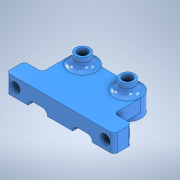
# Autodesk Inventor part: 4mm_Roller_Spacer
Saved by Autodesk Inventor 2021 (Build 250183000, 183)
## iProperties
Created: 2021-03-29
Part Number: 4mm_Roller_Spacer
Material: PET Plastic
Document SubType Name: Modeling
Designer: Jorian Brusind
Density: 1.541 g/cm^3
Appearance: Cyan
Author: Jorian Brusind
Autodesk Inventor part; units mm, degrees
ref_plane "YZ Plane" through (0, 0, 0) normal (1, 0, 0) x (0, 1, 0)
ref_plane "XZ Plane" through (0, 0, 0) normal (0, 1, 0) x (-1, 0, 0)
ref_plane "XY Plane" through (0, 0, 0) normal (0, 0, 1) x (1, 0, 0)
sketch "Sketch4" plane through (0, 0, 0) normal (0, 1, 0) x (-1, 0, 0)
  circle A0 centre (0, 0) radius 7.5
  circle A1 centre (0, 0) radius 2.75
  dimension "d19" = 15
  dimension "d20" = 5.5
  constraints: 2 centre point, 2 coincident
  measures "d19" diameter of A0
  measures "d20" diameter of A1
extrude "Extrusion4" add sketch "Sketch4" along normal blind 10
ref_plane "Work Plane2" through (0, 5, 0) normal (0, 1, 0) x (1, 0, 0)
sketch "Sketch12" plane through (0, 5, 0) normal (0, 1, 0) x (1, 0, 0)
  circle A0 centre (0, 0) radius 2.75 projected
  line L0 (0, 0) -> (25, 0)
  circle A1 centre (25, 0) radius 2.75
  circle A2 centre (25, 0) radius 7.5
  line L1 (12.5, 0) -> (12.5, -20)
  line L2 (42.5, -25) -> (-17.5, -25)
  line L3 (-17.5, -25) -> (-17.5, -15)
  line L4 (-17.5, -15) -> (42.5, -15)
  line L5 (42.5, -15) -> (42.5, -25)
  line L6 (42.5, -25) -> (-17.5, -15) construction
  line L7 (-17.5, -25) -> (42.5, -15) construction
  circle A3 centre (0, 0) radius 7.5 projected
  line L8 (18.6557, -4) -> (6.3443, -4)
  line L9 (6.3443, -4) -> (6.3443, 4)
  line L10 (6.3443, 4) -> (18.6557, 4)
  line L11 (18.6557, 4) -> (18.6557, -4)
  line L12 (18.6557, -4) -> (6.3443, 4) construction
  line L13 (6.3443, -4) -> (18.6557, 4) construction
  line L14 (6.3443, 4) -> (18.6557, 4)
  line L15 (18.6557, 4) -> (18.6557, -16)
  line L16 (18.6557, -16) -> (6.3443, -16)
  line L17 (6.3443, -16) -> (6.3443, 4)
  point P0 (6.3443, -15)
  point P1 (18.6557, -15)
  dimension "d66" = 25
  dimension "d67" = 5.5
  dimension "d68" = 15
  dimension "d69" = 20
  dimension "d70" = 60
  dimension "d71" = 10
  dimension "d72" = 8
  dimension "d73" = 20
  constraints: 36 end point, 6 parallel, 5 midpoint, 4 horizontal, 3 perpendicular, 2 centre point, 2 coincident, 1 vertical, 2 other
  measures "d66" distance of L0.start L0.end
  measures "d67" diameter of A1
  measures "d68" diameter of A2
  measures "d69" distance of L1.start L1.end
  measures "d70" distance of L3.end L4.end
  measures "d71" distance of L2.end L3.end
  measures "d72" distance of L8.end L9.end
  measures "d73" distance of L14.end L15.end
extrude "Extrusion10" add sketch "Sketch12" along normal mid plane 10 contours A3 L10 A2 L0 | L0 L1 L8 A3 | L0 A2 L8 L1 | L8 L1 L4 L17 | A2 L11 L0 | L0 L11 A2 | L8 L15 L4 L1 | A2 L11 | L17 L16 L15 L4 L5 L2 L3 | L4 L1 L16 L17 | L4 L15 L16 L1
sketch "Sketch13" plane through (18.6557, 10, -4) normal (0, 0, -1) x (-1, 0, 0)
  line L0 (36.1557, -10) -> (36.1557, 0) projected
  line L1 (36.1557, -5) -> (31.1557, -5)
  line L2 (31.1557, -9.6188) -> (27.1557, -7.3094)
  line L3 (27.1557, -7.3094) -> (27.1557, -2.6906)
  line L4 (27.1557, -2.6906) -> (31.1557, -0.3812)
  line L5 (31.1557, -0.3812) -> (35.1557, -2.6906)
  line L6 (35.1557, -2.6906) -> (35.1557, -7.3094)
  line L7 (35.1557, -7.3094) -> (31.1557, -9.6188)
  line L8 (-23.8443, -10) -> (-23.8443, 0) projected
  line L9 (-23.8443, -5) -> (-18.8443, -5)
  line L10 (-23.8443, -5) -> (-18.8443, -5) construction
  line L11 (-18.8443, -9.6188) -> (-22.8443, -7.3094)
  line L12 (-22.8443, -7.3094) -> (-22.8443, -2.6906)
  line L13 (-22.8443, -2.6906) -> (-18.8443, -0.3812)
  line L14 (-18.8443, -0.3812) -> (-14.8443, -2.6906)
  line L15 (-14.8443, -2.6906) -> (-14.8443, -7.3094)
  line L16 (-14.8443, -7.3094) -> (-18.8443, -9.6188)
  point P0 (18.6557, -10)
  dimension "d78" = 5
  dimension "d79" = 8
  dimension "d80" = 5
  dimension "d81" = 0
  dimension "d82" = 8
  constraints: 30 end point, 3 horizontal, 2 coincident, 2 midpoint, 1 collinear, 1 parallel, 26 other
  measures "d78" distance of L1.start L1.end
  measures "d79" distance between parallel lines of L3 L6
  measures "d80" distance of L9.start L9.end
  measures "d81" distance between parallel lines of L9 L10
  measures "d82" distance between parallel lines of L12 L15
extrude "Extrusion11" cut sketch "Sketch13" against normal blind 23
fillet "Fillet4" radius 2 8 edges at (18.6557, 5, 15) (6.3443, 5, 15) (-17.5, 5, 25) (42.5, 5, 25) (6.3443, 5, -4) (18.6557, 5, -4) (18.6557, 5, 4) (6.3443, 5, 4)
sketch "Sketch14" plane through (17.6345, 0, -4) normal (0, 0, -1) x (-1, 0, 0)
  circle A0 centre (-19.8655, 5) radius 2.75
  circle A1 centre (30.1345, 5) radius 2.75
  line L0 (35.1345, 0) -> (35.1345, 10) projected
  line L1 (-24.8655, 0) -> (-24.8655, 10) projected
  point P0 (17.6345, 0)
  dimension "d89" = 5.5
  dimension "d90" = 5.5
  dimension "d91" = 5
  dimension "d92" = 5
  constraints: 2 centre point
  measures "d89" diameter of A0
  measures "d90" diameter of A1
  measures "d91" distance from line of L0 A1.centre
  measures "d92" distance from line of L1 A0.centre
extrude "Extrusion12" cut sketch "Sketch14" against normal through all
sketch "Sketch15" plane through (0, 10, 0) normal (0, 1, 0) x (1, 0, 0)
  circle A0 centre (0, 0) radius 2.75
  circle A1 centre (25, 0) radius 2.75 projected
  circle A2 centre (25, 0) radius 2.75
  circle A3 centre (0, 0) radius 2.75 projected
  circle A4 centre (0, 0) radius 4
  circle A5 centre (25, 0) radius 4
  dimension "d95" = 5.5
  dimension "d96" = 5.5
  dimension "d97" = 8
  dimension "d98" = 8
  constraints: 4 centre point, 4 coincident
  measures "d95" diameter of A0
  measures "d96" diameter of A2
  measures "d97" diameter of A4
  measures "d98" diameter of A5
extrude "Extrusion13" add sketch "Sketch15" along normal blind 6
sketch "Sketch17" plane through (0, 0, 0) normal (0, -1, 0) x (1, 0, 0)
  circle A0 centre (0, 0) radius 2.75 projected
  line L0 (0, 0) -> (0, 15)
  line L1 (4.3443, 15) -> (-17.5, 15) projected
  line L2 (0, 15) -> (0, 20)
  line L3 (0, 20) -> (25, 20)
  line L4 (20.6557, 15) -> (42.5, 15) projected
  line L5 (5.5, 25.5) -> (-5.5, 25.5)
  line L6 (-5.5, 25.5) -> (-5.5, 14.5)
  line L7 (-5.5, 14.5) -> (5.5, 14.5)
  line L8 (5.5, 14.5) -> (5.5, 25.5)
  line L9 (5.5, 25.5) -> (-5.5, 14.5) construction
  line L10 (-5.5, 25.5) -> (5.5, 14.5) construction
  line L11 (19.5, 25.5) -> (30.5, 25.5)
  line L12 (30.5, 25.5) -> (30.5, 14.5)
  line L13 (30.5, 14.5) -> (19.5, 14.5)
  line L14 (19.5, 14.5) -> (19.5, 25.5)
  line L15 (19.5, 25.5) -> (30.5, 14.5) construction
  line L16 (30.5, 25.5) -> (19.5, 14.5) construction
  point P0 (30.5, 15)
  point P1 (-5.5, 15)
  point P2 (0, 14.5)
  dimension "d106" = 15
  dimension "d107" = 5
  dimension "d108" = 25
  dimension "d110" = 11
  dimension "d111" = 11
  dimension "d114" = 11
  dimension "d115" = 11
  constraints: 30 end point, 4 midpoint, 4 parallel, 3 horizontal, 2 perpendicular, 2 point on line, 1 vertical
  measures "d106" distance of L0.start L0.end
  measures "d107" distance of L0.end L2.end
  measures "d108" distance of L2.end L3.end
  measures "d110" distance of L7.end L6.end
  measures "d111" distance of L6.end L5.end
  measures "d114" distance of L12.end L13.end
  measures "d115" distance of L11.end L12.end
extrude "Extrusion16" cut sketch "Sketch17" against normal blind 3 contours L0 L2 L3 L8 L7 | L1 L6 L5 L8 L3 L2 | L11 L12 L13 L14
fillet "Fillet5" radius 3 4 edges at (19.5, 3, 19.8161) (30.5, 3, 20) (-5.5, 3, 20) (5.5, 3, 19.8161)
sketch "Sketch18" plane through (0, 10, 0) normal (0, 1, 0) x (1, 0, 0)
  arc A0 (5.8148, 4.7368) -> (3.4297, -6.6699) centre (0, 0) ccw projected
  line L0 (4.3443, -15) -> (-17.5, -15) projected
  line L1 (-7.5, 0) -> (12.5, 0)
  line L2 (-7.5, 0) -> (12.5, 0) construction
  line L3 (-7.5, 0) -> (-7.5, -3)
  line L4 (30.5, -25) -> (30.5, -15) projected
  line L5 (-7.5, -3) -> (32.5, -3)
  circle A1 centre (0, 0) radius 4 projected
  line L6 (-7.5, -3) -> (-7.5, -15)
  line L7 (-7.5, -15) -> (32.5, -15)
  line L8 (42.5, -15) -> (20.6557, -15) projected
  line L9 (32.5, -15) -> (32.5, -3)
  circle A2 centre (25, 0) radius 4 projected
  line L10 (29, 0) -> (32.5, 0)
  arc A3 (21.5703, -6.6699) -> (19.1852, 4.7368) centre (25, 0) ccw projected
  line L11 (32.5, 0) -> (32.5, -3)
  arc A4 (27.6458, -3) -> (29, 0) centre (25, 0) ccw
  arc A5 (-4, 0) -> (-2.6458, -3) centre (0, 0) ccw
  point P0 (22.3542, -3)
  point P1 (2.6458, -3)
  point P2 (-4, 0)
  dimension "d119" = 20
  dimension "d120" = 0
  dimension "d121" = 3
  dimension "d128" = 40
  dimension "d129" = 12
  dimension "d130" = 40
  constraints: 18 end point, 9 point on circle, 6 point on line, 3 horizontal, 2 centre point, 2 coincident, 2 perpendicular, 1 collinear, 1 vertical
  measures "d119" distance of L1.start L1.end
  measures "d120" distance between parallel lines of L1 L2
  measures "d121" distance of L1.start L3.end
  measures "d128" distance of L3.end L5.end
  measures "d129" distance of L3.end L6.end
  measures "d130" distance of L6.end L7.end
extrude "Extrusion18" add sketch "Sketch18" against normal blind 7 contours L1 A1 L5 A0 | A0 L5 L3 | L5 A1 A2 L9 L7 L0 L6 | A2 L10 A3 L5 | A3 L11 L5
fillet "Fillet10" radius 2 4 edges at (-7.5, 6.5, 15) (-17.5, 5, 15) (32.5, 6.5, 15) (42.5, 5, 15)
fillet "Fillet11" radius 3.5 2 edges at (-4, 10, 0) (21, 10, 0)
body "Solid2"
